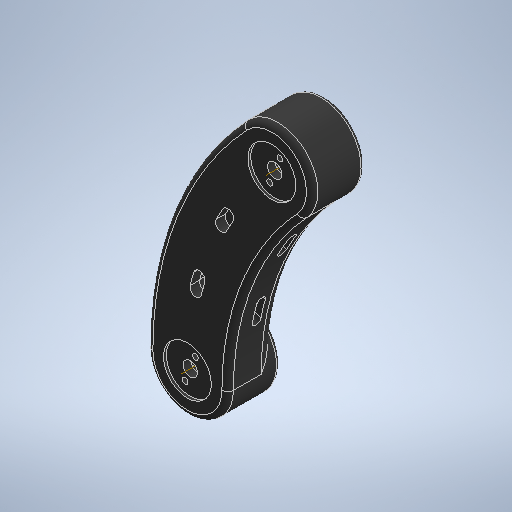
# Autodesk Inventor part: BracoRobotico_0002_002
Saved by Autodesk Inventor 2025.1 (Build 291241020, 241B)
## iProperties
Created: 2025-05-22
Part Number: BracoRobotico_0002_002
Material: Rubber
Document SubType Name: Modeling
Designer: I
Density: 0.93 g/cm^3
Appearance: Rubber - Black
Author: I
Autodesk Inventor part; units mm, degrees
sketch "Sketch2" plane through (0, 0, 0) normal (0, 0, 1) x (1, 0, 0)
  circle A0 centre (0, 0) radius 21 construction
  line L0 (0, 0) -> (21, 0) construction
  circle A1 centre (44.064, 111.617) radius 21 construction
  line L1 (44.064, 111.617) -> (65.064, 111.617) construction
  arc A2 (28.7271, 125.962) -> (-21, 0) centre (163.3986, 0) ccw
  line L2 (-21, 0) -> (0, 0) construction
  arc A3 (59.4009, 97.272) -> (21, 0) centre (163.3986, 0) ccw
  arc A4 (59.4009, 97.272) -> (28.7271, 125.962) centre (44.064, 111.617) ccw
  arc A5 (-21, 0) -> (21, 0) centre (0, 0) ccw
  circle A6 centre (0, 0) radius 120 construction
  line L3 (44.064, 111.617) -> (0, 0) construction
  line L4 (0, 0) -> (0, 120) construction
  arc A7 (21, 0) -> (-21, 0) centre (0, 0) ccw
  arc A8 (28.7271, 125.962) -> (59.4009, 97.272) centre (44.064, 111.617) ccw
  point P0 (0, 21)
  point P1 (29.719, 96.2801)
  point P2 (21, 0)
  dimension "d26" = 42
  dimension "d146" = 239.9999
  dimension "d147" = 21.543
  constraints: 22 point on circle, 10 end point, 9 centre point, 7 coincident, 4 tangent, 3 horizontal, 1 concentric, 1 equal radius, 1 vertical
  measures "d26" diameter of A0
  measures "d146" diameter of A6
  measures "d147" angle of L3 L4
extrude "Extrusion6" add sketch "Sketch2" along normal blind 13.75 and the other way blind 10.75 contours A8 A3 A7 A2
shell "Shell1" thickness 5 removed faces 0
chamfer "Chamfer1" distance 5 angle 45 8 edges at (-3.4676, 65.8752, -5.75) (26.297, 54.1248, -5.75) (27.5308, 91.5508, -5.75) (1.6325, 25.9487, -5.75) (-3.4676, 65.8752, 8.75) (1.6325, 25.9487, 8.75) (26.297, 54.1248, 8.75) (27.5308, 91.5508, 8.75)
sketch "Sketch13" plane through (0, 0, 13.75) normal (0, 0, 1) x (1, 0, 0)
  arc A0 (24.9806, 87.187) -> (2.7509, 30.8777) centre (163.3986, 0) ccw construction
  line L0 (1.1831, 64.0392) -> (21.2934, 56.1001) construction
  circle A1 centre (4.359, 38.3084) radius 3 construction
  line L1 (163.3986, 0) -> (4.359, 38.3084) construction
  line L2 (163.3986, 0) -> (11.2383, 60.0696) construction
  line L3 (163.3986, 0) -> (21.0792, 80.6617) construction
  circle A2 centre (21.0792, 80.6617) radius 3 construction
  arc A3 (6.1814, 45.2092) -> (4.359, 38.3084) centre (163.3986, 0) ccw construction
  arc A4 (3.2982, 46.0382) -> (1.4424, 39.0109) centre (163.3986, 0) ccw
  arc A5 (9.0645, 44.3801) -> (7.2756, 37.6059) centre (163.3986, 0) ccw
  arc A6 (9.0645, 44.3801) -> (3.2982, 46.0382) centre (6.1814, 45.2092) ccw
  arc A7 (1.4424, 39.0109) -> (7.2756, 37.6059) centre (4.359, 38.3084) ccw
  line L4 (6.1814, 45.2092) -> (163.3986, 0) construction
  arc A8 (21.0792, 80.6617) -> (17.6962, 74.377) centre (163.3986, 0) ccw construction
  arc A9 (18.4692, 82.1409) -> (15.0242, 75.741) centre (163.3986, 0) ccw
  arc A10 (23.6891, 79.1824) -> (20.3682, 73.013) centre (163.3986, 0) ccw
  arc A11 (23.6891, 79.1824) -> (18.4692, 82.1409) centre (21.0792, 80.6617) ccw
  arc A12 (15.0242, 75.741) -> (20.3682, 73.013) centre (17.6962, 74.377) ccw
  line L5 (163.3986, 0) -> (17.6962, 74.377) construction
  arc A13 (17.5296, 95.5882) -> (34.9356, 81.9915) centre (44.064, 111.617) ccw construction
  arc A14 (34.9356, 81.9915) -> (13.5704, 27.8719) centre (163.3986, 0) ccw construction
  arc A15 (13.5704, 27.8719) -> (-8.4296, 29.8319) centre (0, 0) ccw construction
  arc A16 (17.5296, 95.5882) -> (-8.4296, 29.8319) centre (163.3986, 0) ccw construction
  point P0 (5.2326, 41.7687)
  dimension "d136" = 6
  dimension "d141" = 8
  dimension "d144" = 2.5
  dimension "d145" = 2.5
  constraints: 31 point on circle, 13 centre point, 12 end point, 8 tangent, 3 coincident, 3 equal radius, 1 concentric, 1 line through centre, 1 midpoint, 1 other
  measures "d136" diameter of A1
  measures "d141" angle of L2 L1
  measures "d144" angle of L4 L1
  measures "d145" angle of L3 L5
extrude "Extrusion9" cut sketch "Sketch13" along normal through all both and the other way through all
extrude "Extrusion1" add sketch "Sketch2" along normal mid plane 27.5 contours A4 A8 | A7 A5
sketch "Sketch3" plane through (0, 0, 13.75) normal (0, 0, 1) x (1, 0, 0)
  circle A0 centre (0, 0) radius 12.5
  arc A1 (55.9522, 94.306) -> (23.2168, 114.146) centre (44.064, 111.617) ccw construction
  arc A2 (55.9522, 94.306) -> (23.2168, 114.146) centre (44.064, 111.617) ccw projected
  circle A3 centre (44.064, 111.617) radius 12.5
  dimension "d53" = 25
  constraints: 2 centre point, 2 coincident, 1 equal radius
  measures "d53" diameter of A0
extrude "Extrusion2" cut sketch "Sketch3" against normal blind 1.5
sketch "Sketch4" plane through (0, 0, 12.25) normal (0, 0, 1) x (1, 0, 0)
  circle A0 centre (0, 0) radius 3.75
  circle A1 centre (2.6618, 6.7437) radius 1.5
  circle A2 centre (-2.6618, -6.7437) radius 1.5
  line L0 (-2.6618, -6.7437) -> (2.6618, 6.7437) construction
  line L1 (0, 0) -> (0, -3.75) construction
  circle A3 centre (44.064, 111.617) radius 12.5 construction
  circle A4 centre (44.064, 111.617) radius 3.75
  circle A5 centre (46.7258, 118.3607) radius 1.5
  circle A6 centre (41.4022, 104.8733) radius 1.5
  line L2 (41.4022, 104.8733) -> (46.7258, 118.3607) construction
  line L3 (44.064, 111.617) -> (44.064, 107.867) construction
  dimension "d56" = 7.5
  dimension "d57" = 14.5
  dimension "d58" = 3
  dimension "d61" = 21.54
  dimension "d106" = 21.54
  constraints: 8 end point, 4 centre point, 4 coincident, 3 equal radius, 3 vertical alignment, 2 midpoint, 1 parallel, 1 vertical, 4 other
  measures "d57" distance of L0.start L0.end
  measures "d58" diameter of A1
  measures "d61" angle of L0 L1
  measures "d106" angle of L2 L3
extrude "Extrusion3" cut sketch "Sketch4" against normal through all
sketch "Sketch5" plane through (0, 0, -13.75) normal (0, 0, -1) x (-1, 0, 0)
  circle A0 centre (0, 0) radius 16
  circle A1 centre (-44.064, 111.617) radius 16
  circle A2 centre (-44.064, 111.617) radius 3.75 construction
  dimension "d64" = 32
  constraints: 2 centre point, 2 coincident, 1 equal radius
  measures "d64" diameter of A0
extrude "Extrusion4" cut sketch "Sketch5" against normal blind 1
sketch "Sketch6" plane through (0, 0, 0) normal (1, 0, 0) x (0, 1, 0)
  circle A0 centre (0, -15.75) radius 16 construction
  line L0 (16, -12.75) -> (-16, -12.75) construction
  line L1 (0, -31.75) -> (0, 0.25)
  arc A1 (0, -31.75) -> (0, 0.25) centre (0, -15.75) ccw
  line L2 (0, 0.25) -> (0, -12.75)
  point P0 (0, 0)
  dimension "d67" = 32
  dimension "d70" = 13
  constraints: 4 end point, 4 point on circle, 2 centre point, 2 midpoint, 1 coincident, 1 collinear, 1 concentric, 1 vertical, 1 vertical alignment
  measures "d67" diameter of A0
  measures "d70" distance of L1.end L2.end
revolve "Revolution1" cut sketch "Sketch6" angle 360 about axis through (0, 0, -31.75) along (0, 0, 1)
ref_plane "Work Plane1" through (44.064, 0, 0) normal (1, 0, 0) x (0, 1, 0)
sketch "Sketch8" plane through (44.064, 0, 0) normal (1, 0, 0) x (0, 1, 0)
  circle A0 centre (111.617, -15.75) radius 16 construction
  line L0 (111.617, -31.75) -> (111.617, 0.25)
  arc A1 (111.617, -31.75) -> (111.617, 0.25) centre (111.617, -15.75) ccw
  line L1 (111.617, 0.25) -> (111.617, -12.75)
  line L2 (107.867, -12.75) -> (115.367, -12.75) construction
  line L3 (107.867, 12.25) -> (115.367, 12.25) construction
  point P0 (0, 0)
  point P1 (111.617, -12.75)
  dimension "d108" = 32
  dimension "d109" = 13
  constraints: 4 end point, 4 point on circle, 3 coincident, 3 midpoint, 2 centre point, 1 collinear, 1 concentric, 1 point on line, 1 vertical
  measures "d108" diameter of A0
  measures "d109" distance of L0.end L1.end
revolve "Revolution2" cut sketch "Sketch8" angle 360 about axis through (44.064, 111.617, -31.75) along (0, 0, 1)
sketch "Sketch7" plane through (0, 0, -13.75) normal (0, 0, -1) x (-1, 0, 0)
  circle A0 centre (0, 0) radius 3.75 construction
  line L0 (2.6618, -6.7437) -> (-2.6618, 6.7437) construction
  line L1 (6.1499, -5.3669) -> (0.8263, 8.1205)
  line L2 (-6.1499, 5.3669) -> (-0.8263, -8.1205)
  arc A1 (-0.8263, -8.1205) -> (6.1499, -5.3669) centre (2.6618, -6.7437) ccw
  arc A2 (0.8263, 8.1205) -> (-6.1499, 5.3669) centre (-2.6618, 6.7437) ccw
  circle A3 centre (-2.6618, 6.7437) radius 1.5 construction
  circle A4 centre (-46.7258, 118.3607) radius 1.5 construction
  circle A5 centre (-44.064, 111.617) radius 3.75 construction
  line L3 (-41.4022, 104.8733) -> (-46.7258, 118.3607) construction
  line L4 (-44.8903, 103.4965) -> (-50.2139, 116.9839)
  line L5 (-43.2377, 119.7375) -> (-37.9141, 106.2501)
  arc A6 (-44.8903, 103.4965) -> (-37.9141, 106.2501) centre (-41.4022, 104.8733) ccw
  arc A7 (-43.2377, 119.7375) -> (-50.2139, 116.9839) centre (-46.7258, 118.3607) ccw
  constraints: 16 end point, 10 tangent, 8 point on circle, 4 centre point, 3 parallel, 2 midpoint, 1 coincident, 1 equal radius
extrude "Extrusion5" cut sketch "Sketch7" against normal blind 22
ref_plane "Work Plane2" through (0, 0, 12.25) normal (0.930142, -0.3672001, 0) x (0, 0, -1)
sketch "Sketch14" plane through (0, 0, 12.25) normal (0.930142, -0.3672001, 0) x (0, 0, -1)
  line L0 (13, 105.4653) -> (13, 14.5347) construction
  line L1 (8.5, 14.5347) -> (8.5, 105.4653) construction
  line L2 (10.75, 85) -> (10.75, 75) construction
  line L3 (8.5, 85) -> (8.5, 75)
  line L4 (13, 75) -> (13, 85)
  arc A0 (13, 85) -> (8.5, 85) centre (10.75, 85) ccw
  arc A1 (8.5, 75) -> (13, 75) centre (10.75, 75) ccw
  line L5 (10.75, 45) -> (10.75, 35) construction
  line L6 (8.5, 45) -> (8.5, 35)
  line L7 (13, 35) -> (13, 45)
  arc A2 (13, 45) -> (8.5, 45) centre (10.75, 45) ccw
  arc A3 (8.5, 35) -> (13, 35) centre (10.75, 35) ccw
  line L8 (10.75, 40) -> (10.75, 80) construction
  point P0 (12.25, 0)
  point P1 (13, 80)
  point P2 (8.5, 80)
  point P3 (13, 40)
  point P4 (8.5, 40)
  point P5 (10.75, 60)
  dimension "d149" = 10
  dimension "d151" = 40
  dimension "d152" = 60
  constraints: 18 end point, 8 point on circle, 8 tangent, 7 midpoint, 4 centre point, 4 point on line, 2 coincident, 2 collinear, 2 parallel, 1 equal radius
  measures "d149" distance of L2.start L2.end
  measures "d151" distance of L8.start L8.end
  measures "d152" vertical distance of point (12.25, 0) point (10.75, 60)
extrude "Extrusion10" cut sketch "Sketch14" along normal through all both and the other way through all
fillet "Fillet2" radius 7 2 edges at (30.9477, 52.2888, -10.75) (-8.1183, 67.7112, -10.75)
fillet "Fillet3" radius 3 4 edges at (58.409, 126.9539, 13.75) (-8.1183, 67.7112, 13.75) (0, -21, 13.75) (30.9477, 52.2888, 13.75)
fillet "Fillet4" radius 2 2 edges at (-21, 0, -13.75) (28.7271, 125.962, -13.75)
body "Solid1"
